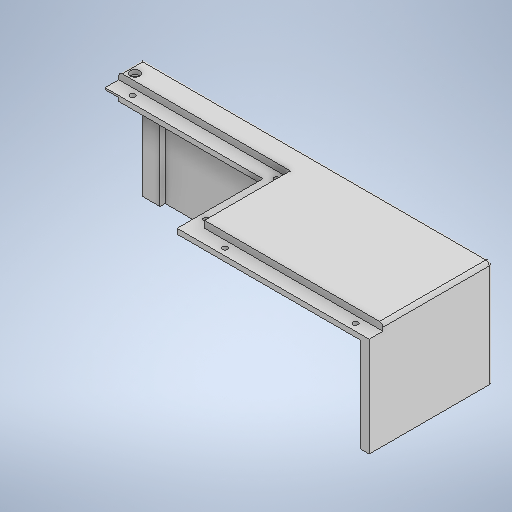
# Autodesk Inventor part: オンゲキボタン_top_right2
Saved by Autodesk Inventor 2025.2 (Build 292293000, 293)
## iProperties
Created: 2025-05-12
Part Number: オンゲキボタン_top_right2
Material: 一般
Document SubType Name: Modeling
Designer: mahhy
Density: 1 g/cm^3
Appearance: 既定
Author: mahhy
## iProperties of the stored document オンゲキボタン_top_right2_3D プリント.ipt
Created: 2025-05-15
Part Number: オンゲキボタン_top_right2_3D プリント
Material: 一般
Document SubType Name: Modeling
Designer: mahhy
Density: 1 g/cm^3
Appearance: 既定
Author: mahhy
Autodesk Inventor part; units mm, degrees
ref_plane "YZ Plane" through (0, 0, 0) normal (1, 0, 0) x (0, 1, 0)
ref_plane "XZ Plane" through (0, 0, 0) normal (0, 1, 0) x (-1, 0, 0)
ref_plane "XY Plane" through (0, 0, 0) normal (0, 0, 1) x (1, 0, 0)
sketch "スケッチ1" plane through (0, 0, 0) normal (0, 1, 0) x (-1, 0, 0)
  line L0 (0, 0) -> (204, 0)
  line L1 (204, 0) -> (204, -72)
  line L2 (204, -72) -> (0, -72)
  line L3 (0, -72) -> (0, 0)
  dimension "d0" = 204
  dimension "d1" = 72
  constraints: 8 end point, 2 parallel, 1 horizontal, 1 perpendicular
  measures "d0" distance of L1.end L2.end
  measures "d1" distance of L0.end L1.end
extrude "押し出し1" add sketch "スケッチ1" along normal blind 7
sketch "スケッチ2" plane through (0, 7, 0) normal (0, 1, 0) x (1, 0, 0)
  line L0 (-204, 72) -> (-204, 0) projected
  line L1 (-204, 0) -> (-112, 0)
  line L2 (-112, 0) -> (-112, 50)
  line L3 (-112, 50) -> (-204, 50)
  line L4 (-204, 50) -> (-204, 0)
  point P0 (0, 0)
  dimension "d4" = 92
  dimension "d5" = 50
  constraints: 8 end point, 2 parallel, 1 horizontal, 1 perpendicular
  measures "d4" distance of L3.end L2.end
  measures "d5" distance of L2.end L1.end
extrude "押し出し2" cut sketch "スケッチ2" against normal through all
sketch "スケッチ3" plane through (0, 7, 0) normal (0, 1, 0) x (1, 0, 0)
  line L0 (-112, 0) -> (0, 0) projected
  line L1 (0, 0) -> (0, 72) projected
  line L2 (-112, 0) -> (0, 0)
  line L3 (0, 0) -> (0, 8)
  line L4 (0, 8) -> (-112, 8)
  line L5 (-112, 8) -> (-112, 0)
  line L6 (-112, 0) -> (-104, 0)
  line L7 (-104, 0) -> (-104, 58)
  line L8 (-104, 58) -> (-112, 58)
  line L9 (-112, 58) -> (-112, 0)
  line L10 (-204, 72) -> (-204, 50) projected
  line L11 (-204, 50) -> (-104, 50)
  line L12 (-104, 50) -> (-104, 58)
  line L13 (-104, 58) -> (-204, 58)
  line L14 (-204, 58) -> (-204, 50)
  point P0 (-112, 50)
  point P1 (-112, 8)
  point P2 (-104, 8)
  dimension "d8" = 8
  dimension "d11" = 8
  dimension "d12" = 8
  constraints: 25 end point, 6 parallel, 3 horizontal, 3 perpendicular, 1 point on line
  measures "d8" distance of L3.end L2.end
  measures "d11" distance of L7.end L8.end
  measures "d12" distance of L7.end L11.end
extrude "押し出し3" cut sketch "スケッチ3" against normal blind 4
sketch "スケッチ4" plane through (0, 3, 0) normal (0, 1, 0) x (1, 0, 0)
  circle A0 centre (-192, 54) radius 1.5
  circle A1 centre (-108, 54) radius 1.5
  circle A2 centre (-108, 13) radius 1.5
  circle A3 centre (-12, 4) radius 1.5
  circle A4 centre (-88, 4) radius 1.5
  line L0 (-204, 50) -> (-204, 58) projected
  line L1 (0, 8) -> (0, 0) projected
  line L2 (-112, 0) -> (-112, 50) projected
  point P0 (-204, 54)
  point P1 (-204, 54)
  point P2 (0, 4)
  point P3 (0, 4)
  dimension "d13" = 3
  dimension "d14" = 3
  dimension "d15" = 3
  dimension "d16" = 3
  dimension "d17" = 3
  dimension "d18" = 12
  dimension "d19" = 12
  dimension "d20" = 24
  dimension "d21" = 4
  dimension "d22" = 41
  constraints: 5 centre point, 4 horizontal alignment, 4 midpoint, 1 vertical alignment
  measures "d13" diameter of A0
  measures "d14" diameter of A1
  measures "d15" diameter of A2
  measures "d16" diameter of A3
  measures "d17" diameter of A4
  measures "d18" distance from line of L0 A0.centre
  measures "d19" distance from line of L1 A3.centre
  measures "d20" distance from line of L2 A4.centre
  measures "d21" distance from line of L2 A2.centre
  measures "d22" distance of A1.centre A2.centre
extrude "押し出し4" cut sketch "スケッチ4" against normal through all
sketch "スケッチ5" plane through (0, 0, 0) normal (0, -1, 0) x (1, 0, 0)
  line L0 (-112, -50) -> (-204, -50) projected
  line L1 (0, -72) -> (-204, -72) projected
  line L2 (-204, -50) -> (-196, -50)
  line L3 (-196, -50) -> (-196, -72)
  line L4 (-196, -72) -> (-204, -72)
  line L5 (-204, -72) -> (-204, -50)
  point P0 (0, 0)
  point P1 (-204, -72)
  dimension "d25" = 8
  constraints: 8 end point, 2 parallel, 1 horizontal, 1 perpendicular, 1 point on line
  measures "d25" distance of L3.end L4.end
extrude "押し出し5" cut sketch "スケッチ5" against normal blind 2
sketch "スケッチ6" plane through (0, 0, 0) normal (0, -1, 0) x (1, 0, 0)
  line L0 (0, -72) -> (-204, -72) projected
  line L1 (-196, -50) -> (-196, -72) projected
  line L2 (0, -72) -> (-196, -72)
  line L3 (-196, -72) -> (-196, -67)
  line L4 (-196, -67) -> (0, -67)
  line L5 (0, -67) -> (0, -72)
  line L6 (0, 0) -> (-5, 0)
  line L7 (-5, 0) -> (-5, -72)
  line L8 (-5, -72) -> (0, -72)
  line L9 (0, -72) -> (0, 0)
  point P0 (-5, -67)
  dimension "d28" = 5
  dimension "d29" = 5
  constraints: 16 end point, 4 parallel, 2 horizontal, 2 perpendicular, 2 point on line
  measures "d28" distance of L2.end L3.end
  measures "d29" distance of L8.end L7.end
extrude "押し出し6" add sketch "スケッチ6" along normal blind 55
sketch "スケッチ7" plane through (-196, 0, -67) normal (0, 0, 1) x (1, 0, 0)
  line L0 (0, 2) -> (0, -55) projected
  line L1 (0, 0) -> (191, 0) projected
  line L2 (0, -55) -> (10, -55)
  line L3 (10, -55) -> (10, 0)
  line L4 (10, 0) -> (0, 0)
  line L5 (0, 0) -> (0, -55)
  point P0 (196, 0)
  dimension "d32" = 10
  constraints: 8 end point, 2 parallel, 1 horizontal, 1 perpendicular, 1 point on line
  measures "d32" distance of L4.end L3.end
extrude "押し出し7" add sketch "スケッチ7" along normal blind 3
sketch "スケッチ8" plane through (-196, 2, -72) normal (-1, 0, 0) x (0, 0, 1)
  circle A0 centre (4, -41) radius 1.5
  circle A1 centre (4, -8) radius 1.5
  line L0 (0, -57) -> (8, -57) projected
  line L1 (0, 0) -> (22, 0) projected
  point P0 (72, -2)
  point P1 (4, -57)
  point P2 (4, -57)
  point P3 (4, -57)
  dimension "d35" = 3
  dimension "d36" = 3
  dimension "d37" = 16
  dimension "d38" = 8
  constraints: 3 midpoint, 2 centre point, 2 vertical alignment
  measures "d35" diameter of A0
  measures "d36" diameter of A1
  measures "d37" distance of point (4, -57) A0.centre
  measures "d38" distance from line of L1 A1.centre
extrude "押し出し8" cut sketch "スケッチ8" against normal blind 8
sketch "スケッチ9" plane through (0, -55, 0) normal (0, -1, 0) x (1, 0, 0)
  line L0 (-5, -67) -> (-5, 0) projected
  circle A0 centre (-5, -8) radius 3
  circle A1 centre (-5, -67) radius 3
  line L1 (-186, -67) -> (-5, -67) projected
  circle A2 centre (-101, -67) radius 3
  circle A3 centre (-191, -67) radius 3
  line L2 (0, 0) -> (-5, 0) projected
  dimension "d41" = 6
  dimension "d42" = 6
  dimension "d43" = 6
  dimension "d44" = 6
  dimension "d46" = 96
  dimension "d47" = 90
  dimension "d73" = 8
  constraints: 4 centre point, 3 point on line
  measures "d41" diameter of A0
  measures "d42" diameter of A1
  measures "d43" diameter of A2
  measures "d44" diameter of A3
  measures "d46" distance of L0.start A2.centre
  measures "d47" distance of A3.centre A2.centre
  measures "d73" distance from line of L2 A0.centre
extrude "押し出し9" add sketch "スケッチ9" against normal blind 15
sketch "スケッチ10" plane through (0, -55, 0) normal (0, -1, 0) x (1, 0, 0)
  arc A0 (-5, -5) -> (-5, -11) centre (-5, -8) ccw projected
  circle A1 centre (-5, -8) radius 1.5
  arc A2 (-5, -64) -> (-8, -67) centre (-5, -67) ccw projected
  circle A3 centre (-5, -67) radius 1.5
  arc A4 (-98, -67) -> (-104, -67) centre (-101, -67) ccw projected
  circle A5 centre (-101, -67) radius 1.5
  circle A6 centre (-189, -67) radius 1.5
  line L0 (-186, -67) -> (-186, -64) projected
  line L1 (-196, -64) -> (-186, -64) projected
  dimension "d50" = 3
  dimension "d51" = 3
  dimension "d52" = 3
  dimension "d58" = 3
  dimension "d59" = 3
  dimension "d60" = 3
  constraints: 4 centre point, 3 coincident
  measures "d50" diameter of A1
  measures "d51" diameter of A3
  measures "d52" diameter of A5
  measures "d58" diameter of A6
  measures "d59" distance from line of L0 A6.centre
  measures "d60" distance from line of L1 A6.centre
extrude "押し出し10" cut sketch "スケッチ10" against normal blind 12
sketch "スケッチ11" plane through (0, 7, 0) normal (0, 1, 0) x (1, 0, 0)
  circle A0 centre (-198.5, 62) radius 1.5
  line L0 (-204, 72) -> (-204, 58) projected
  line L1 (0, 72) -> (-204, 72) projected
  line L2 (-204, 58) -> (-104, 58) projected
  point P0 (0, 0)
  dimension "d61" = 3
  dimension "d63" = 5.5
  dimension "d75" = 4
  constraints: 1 centre point
  measures "d61" diameter of A0
  measures "d63" distance from line of L0 A0.centre
  measures "d75" distance from line of L2 A0.centre
extrude "押し出し11" cut sketch "スケッチ11" against normal through all
sketch "スケッチ12" plane through (0, 7, 0) normal (0, 1, 0) x (1, 0, 0)
  circle A0 centre (-198.5, 62) radius 2.8
  circle A1 centre (-198.5, 62) radius 1.5 projected
  point P0 (0, 0)
  dimension "d68" = 5.6
  constraints: 2 coincident, 1 centre point
  measures "d68" diameter of A0
extrude "押し出し12" cut sketch "スケッチ12" against normal blind 2.5 contours A0 | A1
fillet "フィレット1" radius 2 4 edges at (-204, 7, -65) (-102, 7, -72) (0, 7, -40) (0, -24, -72)
